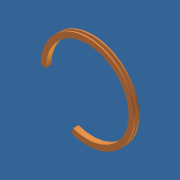
# Autodesk Inventor part: 3510K4
Saved by Autodesk Inventor 2012 SP1 (Build 160190100, 190)
## iProperties
Created: 2012-04-16
Part Number: 3510K4
Material: Default
Vendor: MCMASTER
Document SubType Name: Modeling
Designer: NEGRASHOVI
Density: 1 g/cm^3
Mass: 52.3281 g
Surface Area: 366.42 cm^2
Volume: 52.3281 cm^3
Description: U-channel silicone rubber profile 1/2" x 1/2"
RuleStatus: InUse
AfterDocSave0: file://Part Number Cleaner
SURFACE ROUGHNESS: N/A
SPECIAL FINISH: NONE
ALTERED ITEM PART NUMBER: N/A
ALTERED ITEM VENDOR: N/A
ALTERED ITEM DESCRIPTION: N/A
Author: NEGRASHOVI
Revision Number: 0
Autodesk Inventor part; units mm, degrees
ref_plane "YZ Plane" through (0, 0, 0) normal (1, 0, 0) x (0, 1, 0)
ref_plane "XZ Plane" through (0, 0, 0) normal (0, 1, 0) x (-1, 0, 0)
ref_plane "XY Plane" through (0, 0, 0) normal (0, 0, 1) x (1, 0, 0)
sketch "Sketch1" plane through (0, 0, 0) normal (0, 1, 0) x (-1, 0, 0)
  line L0 (0, 0) -> (0, 6.35)
  line L1 (0, 6.35) -> (12.7, 6.35)
  line L2 (12.7, 6.35) -> (12.7, 3.175)
  line L3 (12.7, 3.175) -> (3.175, 3.175)
  line L4 (15.24, 0) -> (-2.54, 0) construction
  line L5 (3.175, 3.175) -> (3.175, 0)
  line L6 (0, 0) -> (0, -6.35)
  line L7 (0, -6.35) -> (12.7, -6.35)
  line L8 (12.7, -6.35) -> (12.7, -3.175)
  line L9 (12.7, -3.175) -> (3.175, -3.175)
  line L10 (3.175, -3.175) -> (3.175, 0)
  dimension "d0" = 6.35
  dimension "d1" = 3.175
  dimension "d2" = 12.7
  dimension "d3" = 3.175
  constraints: 20 end point, 4 symmetric about line, 3 vertical, 2 horizontal, 1 point on line
  measures "d0" distance of L0.start L0.end
  measures "d1" distance of L1.end L2.end
  measures "d2" distance of L0.end L1.end
  measures "d3" distance between parallel lines of L5 L0
sketch "Sketch2" plane through (0, 0, 0) normal (0, 0, 1) x (1, 0, 0)
  line L0 (-75.0085, 0) -> (283.7112, 0) projected
  arc A0 (63.926, -91.2958) -> (0, 0) centre (97.155, 0) ccw
  line L1 (97.155, 0) -> (63.926, -91.2958) construction
  dimension "d4" = 194.31
  dimension "d6" = 70
  constraints: 2 end point, 2 point on circle, 2 point on line, 1 centre point
  measures "d4" diameter of A0
  measures "d6" angle of L0 L1
sweep "Sweep1" add profiles "Sketch1" path "Sketch2" path curves A0
body "Solid1"
